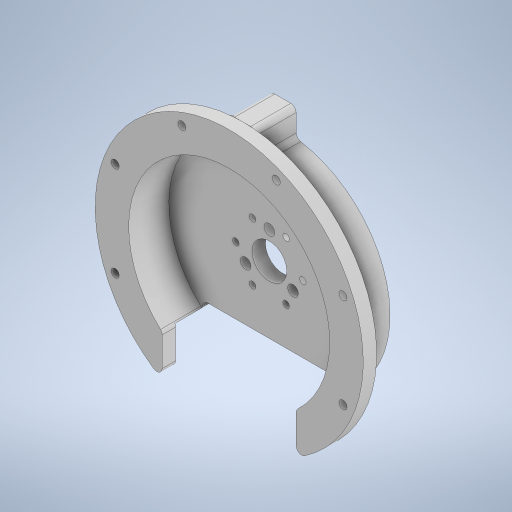
# Autodesk Inventor part: j_r_wy2ky__legparts_01
Saved by Autodesk Inventor 2024.3 (Build 283343000, 343)
## iProperties
Created: 2024-10-20
Part Number: j_r_wy2ky__legparts_01
Material: 一般
Document SubType Name: Modeling
Designer: 佐藤智貴
Density: 1 g/cm^3
Appearance: 既定
Mass: 106.082 g
Surface Area: 211.787 cm^2
Volume: 39.2896 cm^3
Author: 佐藤智貴
Autodesk Inventor part; units mm, degrees
ref_plane "YZ Plane" through (0, 0, 0) normal (1, 0, 0) x (0, 1, 0)
ref_plane "XZ Plane" through (0, 0, 0) normal (0, 1, 0) x (-1, 0, 0)
ref_plane "XY Plane" through (0, 0, 0) normal (0, 0, 1) x (1, 0, 0)
sketch "スケッチ9" plane through (0, 0, 0) normal (0, 0, 1) x (1, 0, 0)
  circle A0 centre (0, 0) radius 40
  dimension "d57" = 80
  constraints: 1 centre point, 1 coincident
  measures "d57" diameter of A0
extrude "押し出し6" add sketch "スケッチ9" along normal blind 15
sketch "スケッチ10" plane through (0, 0, 0) normal (0, 0, -1) x (-1, 0, 0)
  circle A0 centre (0, 0) radius 12.5
  line L0 (0, 0) -> (0, 19.5881)
  line L1 (0, 0) -> (-10.4796, 18.1511)
  point P0 (-6.25, 10.8253)
  point P1 (-12.5, 0)
  point P2 (-6.25, -10.8253)
  point P3 (6.25, -10.8253)
  point P4 (12.5, 0)
  point P5 (6.25, 10.8253)
  dimension "d60" = 25
  dimension "d61" = 30
  dimension "d64" = 360
  constraints: 4 end point, 1 coincident, 1 point on line, 1 vertical, 10 other
  measures "d61" angle of L0 L1
hole "穴4" at (6.25, 10.8253, 0) at (12.5, 0, 0) at (6.25, -10.8253, 0) at (-6.25, -10.8253, 0) at (-12.5, 0, 0) at (-6.25, 10.8253, 0) direction (0, 0, 1) diameter 2.459 end through all
sketch "スケッチ11" plane through (0, 0, 0) normal (0, 0, -1) x (-1, 0, 0)
  circle A0 centre (0, 0) radius 10.2
  point P0 (0, 10.2)
  point P1 (-8.8335, -5.1)
  point P2 (8.8335, -5.1)
  dimension "d73" = 20.4
  dimension "d76" = 360
  constraints: 1 coincident, 1 vertical alignment, 6 other
hole "穴5" at (0, 10.2, 0) at (8.8335, -5.1, 0) at (-8.8335, -5.1, 0) direction (0, 0, 1) diameter 4 end through all
sketch "スケッチ12" plane through (0, 0, 0) normal (0, 0, -1) x (-1, 0, 0)
  circle A0 centre (0, 0) radius 6.5
  dimension "d85" = 13
  constraints: 1 centre point, 1 coincident
  measures "d85" diameter of A0
extrude "押し出し7" cut sketch "スケッチ12" against normal through all
sketch "スケッチ13" plane through (0, 0, 15) normal (0, 0, 1) x (1, 0, 0)
  circle A0 centre (0, 0) radius 50
  dimension "d88" = 100
  constraints: 1 centre point, 1 coincident
  measures "d88" diameter of A0
extrude "押し出し8" add sketch "スケッチ13" along normal blind 5
sketch "スケッチ14" plane through (0, 0, 20) normal (0, 0, 1) x (1, 0, 0)
  circle A0 centre (0, 0) radius 37.5
  dimension "d91" = 75
  constraints: 1 centre point, 1 coincident
  measures "d91" diameter of A0
extrude "押し出し9" cut sketch "スケッチ14" against normal blind 15
sketch "スケッチ15" plane through (0, 0, 20) normal (0, 0, 1) x (1, 0, 0)
  line L0 (0, 0) -> (0, 63.2951)
  circle A0 centre (0, 0) radius 46
  line L1 (0, 0) -> (-20.7267, 50.0386)
  point P0 (-17.6034, 42.4985)
  point P1 (-42.4985, 17.6034)
  point P2 (-42.4985, -17.6034)
  point P3 (-17.6034, -42.4985)
  point P4 (17.6034, -42.4985)
  point P5 (42.4985, -17.6034)
  point P6 (42.4985, 17.6034)
  point P7 (17.6034, 42.4985)
  dimension "d94" = 92
  dimension "d95" = 22.5
  dimension "d98" = 360
  constraints: 4 end point, 1 coincident, 1 point on line, 1 vertical, 12 other
  measures "d95" angle of L0 L1
hole "穴6" at (-17.6034, 42.4985, 20) at (-42.4985, 17.6034, 20) at (-42.4985, -17.6034, 20) at (-17.6034, -42.4985, 20) at (17.6034, -42.4985, 20) at (42.4985, -17.6034, 20) at (42.4985, 17.6034, 20) at (17.6034, 42.4985, 20) direction (0, 0, -1) diameter 3 end through all
sketch "スケッチ16" plane through (0, 0, 20) normal (0, 0, 1) x (1, 0, 0)
  line L0 (-25, -25) -> (25, -25)
  line L1 (25, -25) -> (25, -56.8216)
  line L2 (25, -56.8216) -> (-25, -56.8216)
  line L3 (-25, -56.8216) -> (-25, -25)
  point P0 (0, 0)
  dimension "d107" = 25
  dimension "d108" = 25
  dimension "d109" = 25
  constraints: 8 end point, 2 parallel, 1 horizontal, 1 perpendicular
  measures "d107" distance from line of L3 point (0, 0)
  measures "d108" distance from line of L1 point (0, 0)
  measures "d109" distance from line of L0 point (0, 0)
extrude "押し出し10" cut sketch "スケッチ16" against normal through all
fillet "フィレット2" radius 2 8 edges at (-25, -43.3013, 17.5) (-25, -31.225, 7.5) (-25, -27.9508, 12.5) (-25, -25, 2.5) (25, -43.3013, 17.5) (25, -31.225, 7.5) (25, -27.9508, 12.5) (25, -25, 2.5)
sketch "スケッチ17" plane through (0, 0, 15) normal (0, 0, -1) x (-1, 0, 0)
  arc A0 (28.4211, -28.1468) -> (-28.4211, -28.1468) centre (0, 0) ccw projected
  line L0 (-5, 50) -> (5, 50)
  line L1 (5, 50) -> (5, 39.6863)
  line L2 (5, 39.6863) -> (-5, 39.6863)
  line L3 (-5, 39.6863) -> (-5, 50)
  dimension "d113" = 10
  dimension "d114" = 5
  dimension "d115" = 50
  constraints: 8 end point, 2 parallel, 1 horizontal, 1 perpendicular, 1 point on circle
  measures "d113" distance between parallel lines of L1 L3
  measures "d114" distance from line of point (0, 0) L3
  measures "d115" distance from line of point (0, 0) L0
extrude "押し出し11" add sketch "スケッチ17" along normal blind 15 contours A0 L3 L0 L1
fillet "フィレット3" radius 2 4 edges at (5, 50, 7.5) (5, 39.6863, 7.5) (-5, 39.6863, 7.5) (-5, 50, 7.5)
equation "\"d108\" = d107"
